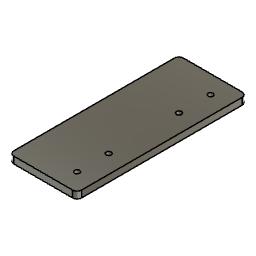
standSide (Autodesk Fusion 360 design; units mm, degrees)
Autodesk Fusion 360 part; units mm, degrees
sketch "Sketch4" plane through (0, 0, 0) normal (0, 0, 1) x (1, 0, 0)
  line L0 (18.9108, 169.079) -> (48.9108, 169.079)
  line L1 (48.9108, 169.079) -> (48.9108, 94.079)
  line L2 (48.9108, 94.079) -> (18.9108, 94.079)
  line L3 (18.9108, 94.079) -> (18.9108, 169.079)
  circle A0 centre (40.9108, 102.079) radius 1.125
  line L4 (48.9108, 109.079) -> (41, 109.079) construction
  circle A1 centre (40.9108, 116.079) radius 1.125
  line L5 (18.9108, 169.079) -> (48.9108, 94.079) construction
  line L6 (18.9108, 94.079) -> (48.9108, 169.079) construction
  line L7 (33.9108, 131.579) -> (48.9108, 131.579) construction
  circle A2 centre (40.9108, 147.079) radius 1.125
  circle A3 centre (40.9108, 161.079) radius 1.125
  dimension "d38" = 2.25
  dimension "d39" = 8
  dimension "d40" = 8
  dimension "d41" = 75
  dimension "d42" = 30
  dimension "d43" = 7
  constraint horizontal L0
  constraint vertical L1
  constraint horizontal L2
  constraint vertical L3
  constraint coincident L1 L4.start
  constraint perpendicular L1 L4
  constraint symmetric A0 L4 A1
  constraint midpoint L5 L7.start
  constraint midpoint L1 L7.end
  constraint symmetric A0 L7 A3
  constraint symmetric A1 L7 A2
  measures "d38" diameter of A0
  measures "d39" distance of L2 A0.centre
  measures "d40" distance of L1 A0.centre
  measures "d41" distance of L0.end L1.end
  measures "d42" distance of L1.end L2.end
  measures "d43" distance of A0.centre L4
extrude "Extrude4" add sketch "Sketch4" along normal blind 3
fillet "Fillet5" radius 2 4 edges at (48.9108, 94.079, 1.5) (18.9108, 94.079, 1.5) (18.9108, 169.079, 1.5) (48.9108, 169.079, 1.5)
